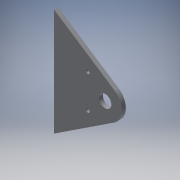
# Autodesk Inventor part: Bearing lockers
Saved by Autodesk Inventor 2018 (Build 220112000, 112)
## iProperties
Created: 2018-05-02
Part Number: Bearing lockers
Material: Generic
Document SubType Name: Modeling
Designer: Ajith Thomas
Density: 1 g/cm^3
Appearance: Default
Author: Ajith Thomas
Autodesk Inventor part; units mm, degrees
ref_plane "YZ Plane" through (0, 0, 0) normal (1, 0, 0) x (0, 1, 0)
ref_plane "XZ Plane" through (0, 0, 0) normal (0, 1, 0) x (-1, 0, 0)
ref_plane "XY Plane" through (0, 0, 0) normal (0, 0, 1) x (1, 0, 0)
sketch "Sketch1" plane through (0, 0, 0) normal (0, 0, 1) x (1, 0, 0)
  circle A0 centre (21.9255, 0) radius 6.5 construction
  arc A1 (28.8018, -10.4387) -> (28.8018, 10.4387) centre (21.9255, 0) ccw projected
  line L0 (-16.0745, -40) -> (28.8018, -10.4387) projected
  line L1 (28.8018, 10.4387) -> (-16.0745, 40) projected
  line L2 (-16.0745, 40) -> (-16.0745, 17) projected
  line L3 (-16.0745, -17) -> (-16.0745, -40) projected
  line L4 (-16.0745, -40) -> (-16.0745, 40)
  circle A2 centre (21.9255, 0) radius 4.675
  circle A3 centre (8.9255, -12.5) radius 1.5
  line L5 (-16.0745, 0) -> (34.4255, 0) construction
  circle A4 centre (8.9255, 12.5) radius 1.5
  point P0 (0, 0)
  dimension "d0" = 9.35
  dimension "d1" = 3
  dimension "d2" = 25
  dimension "d3" = 12.5
  constraints: 4 end point, 3 centre point, 1 coincident, 1 midpoint, 1 point on circle, 1 symmetric about line, 1 vertical, 1 other
  measures "d0" diameter of A2
  measures "d1" diameter of A3
  measures "d2" distance from line of L4 A3.centre
  measures "d3" distance from line of L5 A3.centre
extrude "Extrusion1" add sketch "Sketch1" along normal blind 3
body "Solid1"
